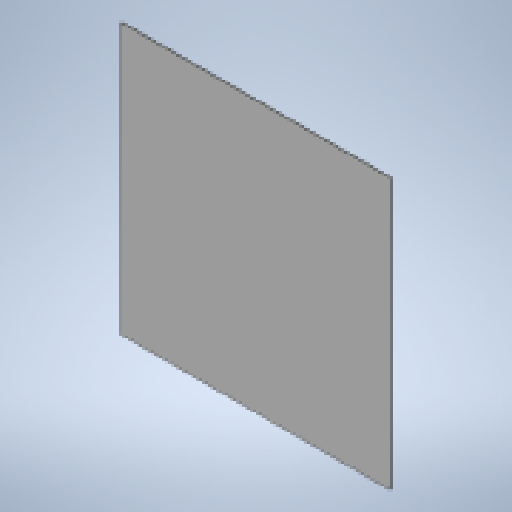
# Autodesk Inventor part: GBK 3339 shield 9
Saved by Autodesk Inventor 2026 (Build 300175000, 175)
## iProperties
Created: 2026-04-17
Part Number: GBK 3339 shield 9
Material: Steel
Document SubType Name: Sheet Metal
Designer: pokla
Stock Number: 3339
Mass: 69243.3 g
Surface Area: 44341.6 cm^2
Volume: 8820.8 cm^3
Density: 7.85 g/cm^3
Flat Pattern Width: 148 cm
Flat Pattern Length: 149 cm
Flat Pattern Area: 22052 cm^2
Sheet Metal Rule: По умолчанию_мм
Sheet Metal Width: 1480,000 мм
Sheet Metal Length: 1490,000 мм
Sheet Metal Area: 2205200,000 мм^2
Appearance: Default
Author: admin
Autodesk Inventor part; units mm, degrees
ref_plane "YZ Plane" through (0, 0, 0) normal (1, 0, 0) x (0, 1, 0)
ref_plane "XZ Plane" through (0, 0, 0) normal (0, 1, 0) x (-1, 0, 0)
ref_plane "XY Plane" through (0, 0, 0) normal (0, 0, 1) x (1, 0, 0)
sketch "Sketch1" plane through (0, 0, 0) normal (0, 0, 1) x (1, 0, 0)
  line L0 (740, -745) -> (-740, -745)
  line L1 (-740, -745) -> (-740, 745)
  line L2 (-740, 745) -> (740, 745)
  line L3 (740, 745) -> (740, -745)
  line L4 (740, -745) -> (-740, 745) construction
  line L5 (-740, -745) -> (740, 745) construction
  point P0 (0, 0)
  dimension "d0" = 1480
  dimension "d1" = 1490
  measures "d0" distance of L1.end L2.end
  measures "d1" distance of L0.end L1.end
extrude "Plate1" add sketch "Sketch1" along normal blind 4
sketch "Эскиз2" plane through (0, 0, 0) normal (0, 0, -1) x (-1, 0, 0)
  line L0 (582.7476, -597.0649) -> (582.7476, -1095.2011) construction
  line L1 (582.7476, -1095.2011) -> (543.1204, -1095.2011) construction
  line L2 (543.1204, -1095.2011) -> (543.1204, -597.0649) construction
  line L3 (543.1204, -597.0649) -> (582.7476, -597.0649) construction
  line L4 (209.363, -591.5) -> (209.363, -494.5) projected
  line L5 (209.363, -591.5) -> (205.363, -591.5) projected
  line L6 (-290.5101, -494.5) -> (-290.5101, -591.5) projected
  line L7 (-290.5101, -591.5) -> (-294.5101, -591.5) projected
  line L8 (209.363, 713.5) -> (209.363, 773.5) projected
  line L9 (209.363, 713.5) -> (205.363, 713.5) projected
  line L10 (-290.5101, 713.5) -> (-290.5101, 773.5) projected
  line L11 (-290.5101, 713.5) -> (-294.5101, 713.5) projected
  line L12 (739.6246, -491) -> (739.6246, -487) projected
  line L13 (739.6246, 5.667) -> (739.6246, 9.667) projected
  line L14 (739.6246, 502.334) -> (739.6246, 506.334) projected
  line L15 (-740, -491) -> (-710, -491) projected
  line L16 (-710, -491) -> (-710, -487) projected
  line L17 (-740, 5.667) -> (-710, 5.667) projected
  line L18 (-710, 5.667) -> (-710, 9.667) projected
  line L19 (-740, 502.334) -> (-710, 502.334) projected
  line L20 (-710, 502.334) -> (-710, 506.334) projected
  line L21 (739.6246, -491) -> (709.6246, -491)
  line L22 (739.6246, 5.6667) -> (709.6246, 5.6667)
  line L23 (739.6246, 502.3333) -> (709.6246, 502.3333)
  point P0 (0, 0)
  dimension "d3" = 30
  dimension "d4" = 30
  dimension "d5" = 30
  constraints: 6 end point, 3 horizontal, 2 other
  measures "d3" distance of L12.start L21.end
  measures "d4" distance of L22.start L22.end
  measures "d5" distance of L23.start L23.end
mark "Маркировка1"
equation "\"d0\" = Лист_ширина"
equation "\"d1\" = 0.5 * Лист_длина"
equation "\"d2\" = Thickness"
equation "\"BendRadius\" = Thickness"
equation "\"BendReliefWidth\" = Thickness"
equation "\"BendReliefDepth\" = 0.5 * Thickness"
equation "\"CornerReliefSize\" = 4 * Thickness"
equation "\"MinimumRemnant\" = 2 * Thickness"
equation "\"TransitionRadius\" = BendRadius"
equation "\"JacobiRadiusSize\" = BendRadius"
equation "\"GapSize\" = Thickness"
equation "\"Лист_ширина\" = 1480"
equation "\"Лист_длина\" = 2980"
equation "\"Thickness\" = 4"
body "Solid1"
